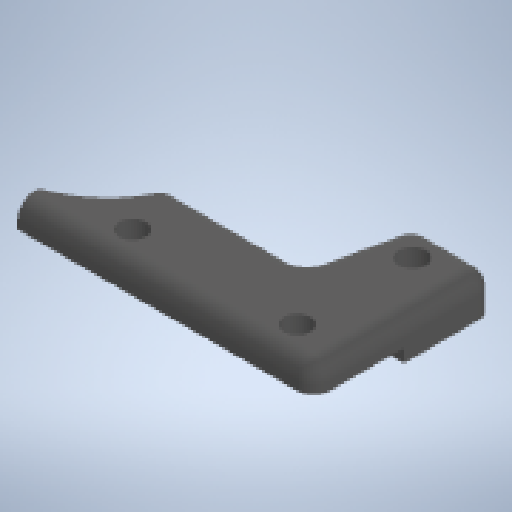
# Autodesk Inventor part: leg_springjoint_cover_under_left
Saved by Autodesk Inventor 2024.1 (Build 281209000, 209)
## iProperties
Created: 2024-02-13
Part Number: leg_springjoint_cover_under_left
Material: 一般
Document SubType Name: Modeling
Designer: hibik
Density: 1 g/cm^3
Appearance: 既定
Author: hibik
Autodesk Inventor part; units mm, degrees
ref_plane "YZ Plane" through (0, 0, 0) normal (1, 0, 0) x (0, 1, 0)
ref_plane "XZ Plane" through (0, 0, 0) normal (0, 1, 0) x (-1, 0, 0)
ref_plane "XY Plane" through (0, 0, 0) normal (0, 0, 1) x (1, 0, 0)
sketch "スケッチ1" plane through (0, 0, 0) normal (0, 1, 0) x (-1, 0, 0)
  line L0 (20, 0) -> (0, 0)
  line L1 (0, 0) -> (0, -27)
  line L2 (0, -27) -> (20, -27)
  line L3 (20, -27) -> (20, 0)
  circle A0 centre (20, -13.5) radius 13.5
  circle A1 centre (20, -13.5) radius 14
  circle A2 centre (20, -13.5) radius 2
  line L4 (20, -11.5) -> (-0.0059, -11.5)
  line L5 (0, -27) -> (20, -27)
  line L6 (20, -27) -> (20, -17)
  line L7 (20, -17) -> (0, -17)
  line L8 (0, -17) -> (0, -27)
  line L9 (20, -11.5) -> (0, -11.5)
  line L10 (0, -11.5) -> (0, -6)
  line L11 (0, -6) -> (20, -6)
  line L12 (20, -6) -> (20, -11.5)
  circle A3 centre (20, -13.5) radius 6.5
  line L13 (20, -10.5) -> (-0.0015, -10.5)
  line L14 (6.3252, -10.5) -> (2.7054, -27)
  point P0 (16.2919, 0)
  point P1 (16.2919, -27)
  point P2 (0, -11.5)
  point P3 (6.1436, -11.5)
  point P4 (0, -17)
  point P5 (6.4446, -17)
  point P6 (8.1784, -6)
  point P7 (13.8153, -11.5)
  point P8 (20, -7)
  point P9 (14.5228, -17)
  point P10 (20, -20)
  point P11 (6.1058, -11.5)
  point P12 (4.8992, -17)
  dimension "d1" = 28
  dimension "d2" = 4
  dimension "d0" = 27
  dimension "d7" = 20
  dimension "d8" = 10
  dimension "d9" = 5.5
  dimension "d21" = 13
  dimension "d22" = 1
  constraints: 30 end point, 7 parallel, 5 point on line, 4 horizontal, 3 coincident, 3 perpendicular, 2 centre point, 2 midpoint, 1 tangent, 1 vertical alignment, 7 other
  measures "d0" diameter of A0
  measures "d7" distance of L0.start L0.end
  measures "d8" distance between parallel lines of L2 L7
  measures "d9" distance between parallel lines of L4 L11
  measures "d21" diameter of A3
  measures "d22" distance between parallel lines of L4 L13
extrude "押し出し1" add sketch "スケッチ1" along normal blind 2.3 contours L3 A3 L13 A0 L11 | A0 L13 A1 L11 | A1 L13 L1 L11 | L13 A3 L4 A0 | A0 L4 A1 L13 | L14 L4 L1 L13 | A1 L4 L14 | L14 L7 L1 L4
extrude "押し出し2" cut sketch "スケッチ1" along normal blind 0.8 contours A1 L11 L1 L0 | L3 A3 L13 A0 L11 | A0 L13 A1 L11 | A1 L13 L1 L11 | L13 A3 L4 A0 | A0 L4 A1 L13 | L14 L4 L1 L13 | A1 L4 L14
sketch "スケッチ2" plane through (0, 2.3, 0) normal (0, 1, 0) x (1, 0, 0)
  circle A0 centre (-3, 15) radius 0.8
  line L0 (-20, 6) -> (0, 6) projected
  line L1 (0, 0) -> (0, 17) projected
  circle A1 centre (-3, 8) radius 0.8
  line L2 (0, 17) -> (-4.8992, 17) projected
  circle A2 centre (-13, 8) radius 0.8
  circle A3 centre (-13, 8) radius 0.8 projected
  circle A4 centre (-3, 8) radius 0.8 projected
  line L3 (-18, 0) -> (-18, 7.3153) projected
  line L4 (-18, 0) -> (0.4606, 0) projected
  line L5 (0.4606, 0.5589) -> (0.4606, 0) projected
  arc A5 (0.4606, 5.4411) -> (0.4606, 0.5589) centre (1, 3) ccw projected
  line L6 (0.4606, 10.5) -> (0.4606, 5.4411) projected
  line L7 (0.4606, 10.5) -> (-14.2337, 10.5) projected
  arc A6 (-18, 7.3153) -> (-14.2337, 10.5) centre (-20, 13.5) ccw projected
  arc A7 (-20, 7) -> (-13.8153, 11.5) centre (-20, 13.5) ccw projected
  line L8 (-20, 7) -> (-20, 6) projected
  line L9 (-20, 6) -> (0, 6) projected
  line L10 (0, 6) -> (0, 17) projected
  line L11 (0, 17) -> (-4.8992, 17) projected
  line L12 (-4.8992, 17) -> (-6.1058, 11.5) projected
  line L13 (-6.1058, 11.5) -> (-13.8153, 11.5) projected
  point P0 (-8.1784, 6)
  point P1 (-6.4446, 17)
  point P2 (-5.3497, 17)
  point P3 (0, 27)
  point P4 (-14.5228, 17)
  point P5 (-20, 17)
  point P6 (-18, 6)
  dimension "d11" = 1.6
  dimension "d14" = 1.6
  dimension "d15" = 2
  dimension "d16" = 3
  dimension "d17" = 2
  dimension "d23" = 1.6
  dimension "d24" = 10
  constraints: 3 centre point, 1 horizontal alignment, 1 vertical alignment
  measures "d11" diameter of A0
  measures "d14" diameter of A1
  measures "d15" distance from line of L0 A1.centre
  measures "d16" distance from line of L1 A1.centre
  measures "d17" distance from line of L2 A0.centre
  measures "d23" diameter of A2
  measures "d24" distance of A1.centre A2.centre
extrude "押し出し3" cut sketch "スケッチ2" against normal through all contours A0 | L8 A7 L3 L0 | A1 | A2
fillet "フィレット1" radius 1 9 edges at (0, 1.55, -6) (0, 1.15, -17) (-9, 2.3, -6) (0, 2.3, -11.5) (-2.4496, 2.3, -17) (-9.9606, 2.3, -11.5) (-5.5025, 2.3, -14.25) (-4.8992, 1.15, -17) (-6.1058, 1.55, -11.5)
